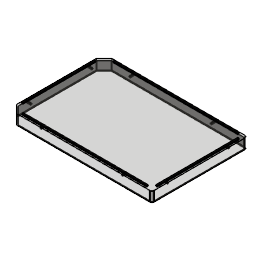
Container V3.4 (Assembly) (Autodesk Fusion 360 archive; units mm, degrees)
design "GREINER 96 WELL PLATE LID"
part number: 2026-02-05-10-27-23-618
Autodesk Fusion 360 part; units mm, degrees
(part 1 of 2)
sketch "Sketch1" plane through (0, 0, 0) normal (0, 0, 1) x (1, 0, 0)
  line L0 (61.42, -42.3) -> (-56.55, -42.3)
  line L1 (-63.55, -35.3) -> (-63.55, 35.3)
  line L2 (-56.55, 42.3) -> (61.42, 42.3)
  line L3 (63.55, 40.17) -> (63.55, -40.17)
  line L4 (63.55, -42.3) -> (-63.55, 42.3) construction
  line L5 (-63.55, -42.3) -> (63.55, 42.3) construction
  line L6 (-56.55, 42.3) -> (-63.55, 35.3)
  line L7 (0, -42.3) -> (0, 42.3) construction
  line L8 (63.55, 0) -> (-63.55, 0) construction
  line L9 (-56.55, -42.3) -> (-63.55, -35.3)
  arc A0 (63.55, 40.17) -> (61.42, 42.3) centre (61.42, 40.17) ccw
  arc A1 (61.42, -42.3) -> (63.55, -40.17) centre (61.42, -40.17) ccw
  dimension "d1" = 84.6
  dimension "d2" = 127.1
  dimension "d3" = 7
  dimension "d4" = 7
  dimension "d5" = 2.13
  constraint horizontal L0
  constraint perpendicular L0 L1
  constraint parallel L0 L2
  constraint parallel L1 L3
  constraint coincident L4 origin
  constraint coincident L5 origin
  constraint coincident L4.end L2
  constraint coincident L4.end L1
  constraint coincident L2 L7.end
  constraint perpendicular L2 L7
  constraint coincident L1 L8.end
  constraint perpendicular L1 L8
  constraint symmetric L2.start L8 L0.end
  constraint symmetric L1.end L8 L1.start
  constraint coincident L0 L7.start
  constraint coincident L3 L8.start
  constraint coincident L5.end L2
  constraint coincident L5.end L3
  constraint tangent L2 A0
  constraint tangent L3 A0
  constraint symmetric L8 L2.end L0.start
  constraint symmetric L8 L3.start L3.end
  constraint symmetric L8 A0 A1
  measures "d1" distance of L5.start L4.end
  measures "d2" distance of L4.end L5.end
  measures "d3" distance of L4.end L2.start
  measures "d4" distance of L4.end L1.end
  measures "d5" radius of A0
extrude "Extrude1" add sketch "Sketch1" against normal blind 9
sketch "Sketch2" plane through (0, 0, -9) normal (0, 0, -1) x (1, 0, 0)
  line L0 (61.42, 42.3) -> (-56.55, 42.3)
  line L1 (-56.55, 42.3) -> (-63.55, 35.3)
  line L2 (-63.55, 35.3) -> (-63.55, -35.3)
  line L3 (-63.55, -35.3) -> (-56.55, -42.3)
  line L4 (-56.55, -42.3) -> (61.42, -42.3)
  arc A0 (61.42, -42.3) -> (63.55, -40.17) centre (61.42, -40.17) ccw
  line L5 (63.55, -40.17) -> (63.55, 40.17)
  arc A1 (63.55, 40.17) -> (61.42, 42.3) centre (61.42, 40.17) ccw
  line L6 (61.42, -41.3) -> (-56.1358, -41.3)
  line L7 (-62.55, -34.8858) -> (-62.55, 34.8858)
  line L8 (-56.1358, 41.3) -> (61.42, 41.3)
  line L9 (62.55, 40.17) -> (62.55, -40.17)
  line L10 (62.55, -41.3) -> (-62.55, 41.3) construction
  line L11 (-62.55, -41.3) -> (62.55, 41.3) construction
  line L12 (-56.1358, 41.3) -> (-62.55, 34.8858)
  arc A2 (62.55, 40.17) -> (61.42, 41.3) centre (61.42, 40.17) ccw
  line L13 (63.55, 0) -> (-63.55, 0) construction
  line L14 (-56.1358, -41.3) -> (-62.55, -34.8858)
  arc A3 (61.42, -41.3) -> (62.55, -40.17) centre (61.42, -40.17) ccw
  dimension "d8" = 125.1
  dimension "d9" = 82.6
  dimension "d10" = 6.4142
  dimension "d11" = 6.4142
  dimension "d12" = 1
  dimension "d13" = 1.13
  constraint horizontal L6
  constraint perpendicular L6 L7
  constraint parallel L6 L8
  constraint parallel L7 L9
  constraint coincident L10 origin
  constraint coincident L11 origin
  constraint coincident L10.end L8
  constraint coincident L10.end L7
  constraint coincident L11.end L9
  constraint coincident L11.end L8
  constraint tangent L9 A2
  constraint tangent L8 A2
  constraint midpoint L5 L13.start
  constraint midpoint L2 L13.end
  constraint symmetric L8.start L13 L6.end
  constraint symmetric L7.end L13 L7.start
  constraint symmetric L9.start L13 L9.end
  constraint symmetric L8.end L13 L6.start
  constraint symmetric A2 L13 A3
  measures "d8" distance of L10.end L11.end
  measures "d9" distance of L11.start L10.end
  measures "d10" distance of L10.end L8.start
  measures "d11" distance of L10.end L7.end
  measures "d12" distance of L1 L12
  measures "d13" radius of A2
extrude "Extrude2" cut sketch "Sketch2" against normal blind 8 contours L6 L7 L8 L9 L12 A2 L14 A3
sketch "Sketch3" plane through (0, 0, -1) normal (0, 0, -1) x (1, 0, 0)
  line L0 (-56.1358, -41.3) -> (61.42, -41.3)
  arc A0 (61.42, -41.3) -> (62.55, -40.17) centre (61.42, -40.17) ccw
  line L1 (62.55, -40.17) -> (62.55, 40.17)
  arc A1 (62.55, 40.17) -> (61.42, 41.3) centre (61.42, 40.17) ccw
  line L2 (61.42, 41.3) -> (-56.1358, 41.3)
  line L3 (-56.1358, 41.3) -> (-62.55, 34.8858)
  line L4 (-62.55, 34.8858) -> (-62.55, -34.8858)
  line L5 (-62.55, -34.8858) -> (-56.1358, -41.3)
  line L6 (-62.55, 32.8642) -> (-35.55, 32.8642) construction
  line L7 (-35.55, 32.8642) -> (-35.55, 41.3) construction
  line L8 (-35.55, 41.3) -> (-36.55, 41.3)
  line L9 (-36.55, 41.3) -> (-36.55, 37.5)
  line L10 (-36.55, 37.5) -> (-35.55, 37.5)
  line L11 (-35.55, 37.5) -> (-35.55, 41.3)
  line L12 (-50.2731, 41.3) -> (-50.2731, 26.6) construction
  line L13 (-50.2731, 26.6) -> (-62.55, 26.6) construction
  line L14 (-62.55, 26.6) -> (-58.75, 26.6)
  line L15 (-58.75, 26.6) -> (-58.75, 27.6)
  line L16 (-58.75, 27.6) -> (-62.55, 27.6)
  line L17 (-62.55, 27.6) -> (-62.55, 26.6)
  line L18 (62.55, 0) -> (-62.55, 0) construction
  line L19 (-62.55, 30.673) -> (-62.55, 55) construction
  line L20 (62.55, 34.8173) -> (62.55, 55) construction
  line L21 (62.55, 55) -> (-62.55, 55) construction
  line L22 (0, 55) -> (0, -41.3) construction
  line L23 (62.55, 27.6) -> (62.55, 26.6)
  line L24 (62.55, 26.6) -> (58.75, 26.6)
  line L25 (58.75, 27.6) -> (62.55, 27.6)
  line L26 (58.75, 26.6) -> (58.75, 27.6)
  line L27 (36.55, 41.3) -> (36.55, 37.5)
  line L28 (35.55, 37.5) -> (35.55, 41.3)
  line L29 (36.55, 37.5) -> (35.55, 37.5)
  line L30 (35.55, 41.3) -> (36.55, 41.3)
  line L31 (62.55, -26.6) -> (58.75, -26.6)
  line L32 (58.75, -27.6) -> (62.55, -27.6)
  line L33 (58.75, -26.6) -> (58.75, -27.6)
  line L34 (35.55, -37.5) -> (35.55, -41.3)
  line L35 (36.55, -37.5) -> (35.55, -37.5)
  line L36 (36.55, -41.3) -> (36.55, -37.5)
  line L37 (62.55, -27.6) -> (62.55, -26.6)
  line L38 (35.55, -41.3) -> (36.55, -41.3)
  line L39 (-58.75, -26.6) -> (-58.75, -27.6)
  line L40 (-62.55, -26.6) -> (-58.75, -26.6)
  line L41 (-58.75, -27.6) -> (-62.55, -27.6)
  line L42 (-62.55, -27.6) -> (-62.55, -26.6)
  line L43 (-36.55, -37.5) -> (-35.55, -37.5)
  line L44 (-35.55, -37.5) -> (-35.55, -41.3)
  line L45 (-36.55, -41.3) -> (-36.55, -37.5)
  line L46 (-35.55, -41.3) -> (-36.55, -41.3)
  dimension "d16" = 27
  dimension "d17" = 3.8
  dimension "d18" = 1
  dimension "d19" = 14.7
  dimension "d20" = 3.8
  dimension "d21" = 1
  constraint coincident L4 L6.start
  constraint perpendicular L4 L6
  constraint coincident L2 L7.end
  constraint perpendicular L2 L7
  constraint horizontal L8
  constraint vertical L9
  constraint horizontal L10
  constraint vertical L11
  constraint coincident L2 L12.start
  constraint perpendicular L2 L12
  constraint coincident L4 L13.end
  constraint perpendicular L4 L13
  constraint horizontal L14
  constraint vertical L15
  constraint horizontal L16
  constraint vertical L17
  constraint midpoint L1 L18.start
  constraint midpoint L4 L18.end
  constraint coincident L4 L19.start
  constraint perpendicular L6 L19
  constraint coincident L1 L20.start
  constraint parallel L1 L20
  constraint perpendicular L19 L21
  constraint midpoint L21 L22.start
  constraint coincident L0 L22.end
  constraint perpendicular L0 L22
  constraint symmetric L7.end L22 L28.end
  constraint symmetric L8.end L22 L27.start
  constraint symmetric L9.end L22 L27.end
  constraint symmetric L10.end L22 L28.start
  constraint symmetric L13.end L22 L23.end
  constraint symmetric L14.end L22 L24.end
  constraint symmetric L15.end L22 L25.start
  constraint symmetric L16.end L22 L23.start
  constraint symmetric L7.end L18 L44.end
  constraint symmetric L8.end L18 L45.start
  constraint symmetric L9.end L18 L43.start
  constraint symmetric L10.end L18 L43.end
  constraint symmetric L13.end L18 L40.start
  constraint symmetric L14.end L18 L39.start
  constraint symmetric L15.end L18 L39.end
  constraint symmetric L16.end L18 L41.end
  constraint symmetric L18 L23.start L32.end
  constraint symmetric L18 L23.end L31.start
  constraint symmetric L18 L27.end L35.start
  constraint symmetric L18 L28.start L34.start
  constraint symmetric L18 L24.end L31.end
  constraint symmetric L18 L25.start L32.start
  constraint symmetric L18 L27.start L36.start
  constraint symmetric L18 L28.end L34.end
  measures "d16" distance of L6.start L6.end
  measures "d17" distance of L8.end L9.end
  measures "d18" distance of L9.end L10.end
  measures "d19" distance of L12.start L12.end
  measures "d20" distance of L15.end L16.end
  measures "d21" distance of L14.end L15.end
extrude "Extrude3" add sketch "Sketch3" along normal blind 1 contours L0 L43 L44 L45 L46 | L4 L39 L40 L41 L42 | L0 L34 L35 L36 L38 | L4 L14 L15 L16 L17 | L1 L31 L32 L33 L37 | L2 L8 L9 L10 L11 | L1 L23 L24 L25 L26 | L2 L27 L28 L29 L30
sketch "Sketch4" plane through (0, 0, 0) normal (0, 0, 1) x (-1, 0, 0)
  line L0 (56.55, 42.3) -> (-61.42, 42.3)
  arc A0 (-61.42, 42.3) -> (-63.55, 40.17) centre (-61.42, 40.17) ccw
  line L1 (-63.55, 40.17) -> (-63.55, -40.17)
  arc A1 (-63.55, -40.17) -> (-61.42, -42.3) centre (-61.42, -40.17) ccw
  line L2 (-61.42, -42.3) -> (56.55, -42.3)
  line L3 (56.55, -42.3) -> (63.55, -35.3)
  line L4 (63.55, -35.3) -> (63.55, 35.3)
  line L5 (63.55, 35.3) -> (56.55, 42.3)
  line L6 (-63.55, -34.3916) -> (-62.25, -34.3916) construction
  line L7 (-62.25, -34.3916) -> (-62.25, -36.4) construction
  line L8 (-60, -42.3) -> (-66.2, -42.3) construction
  line L9 (-63.55, -39.2433) -> (-63.55, -43.1) construction
  line L10 (-62.25, -36.4) -> (-60.95, -36.4)
  line L11 (-60.95, -36.4) -> (-60.95, 36.4)
  line L12 (-60.95, 36.4) -> (-62.25, 36.4)
  line L13 (-62.25, 36.4) -> (-62.25, -36.4)
  line L14 (-52.6219, -42.3) -> (-52.6219, -41) construction
  line L15 (-52.6219, -41) -> (-57.65, -41) construction
  line L16 (-57.65, -41) -> (53.05, -41)
  line L17 (53.05, -41) -> (53.05, -39.7)
  line L18 (53.05, -39.7) -> (-57.65, -39.7)
  line L19 (-57.65, -39.7) -> (-57.65, -41)
  line L20 (53.05, 39.7) -> (-57.65, 39.7)
  line L21 (-57.65, 41) -> (53.05, 41)
  line L22 (-57.65, 39.7) -> (-57.65, 41)
  line L23 (53.05, 41) -> (53.05, 39.7)
  line L24 (60.95, 0) -> (60.95, -32.3)
  line L25 (60.95, -32.3) -> (62.25, -32.3)
  line L26 (62.25, -32.3) -> (62.25, 0)
  line L27 (60.95, 0) -> (60.95, 32.3)
  line L28 (62.25, 32.3) -> (62.25, 0)
  line L29 (60.95, 32.3) -> (62.25, 32.3)
  line L30 (-63.55, 0) -> (60.95, 0) construction
  line L31 (62.25, 0) -> (63.55, 0) construction
  dimension "d24" = 1.3
  dimension "d25" = 5.9
  dimension "d26" = 72.8
  dimension "d27" = 1.3
  dimension "d28" = 1.3
  dimension "d29" = 5.9
  dimension "d30" = 1.3
  dimension "d31" = 110.7
  dimension "d32" = 32.3
  dimension "d33" = 1.3
  dimension "d34" = 1.3
  constraint coincident L1 L6.start
  constraint perpendicular L1 L6
  constraint perpendicular L6 L7
  constraint coincident L2 L8.start
  constraint parallel L2 L8
  constraint coincident L1 L9.start
  constraint perpendicular L2 L9
  constraint horizontal L10
  constraint vertical L11
  constraint horizontal L12
  constraint vertical L13
  constraint coincident L2 L14.start
  constraint perpendicular L2 L14
  constraint perpendicular L14 L15
  constraint horizontal L16
  constraint vertical L17
  constraint horizontal L18
  constraint vertical L19
  constraint midpoint L1 L30.start
  constraint midpoint L4 L31.end
  constraint symmetric L15.end L21.start L30
  constraint symmetric L16.end L21.end L30
  constraint symmetric L17.end L20.start L30
  constraint symmetric L18.end L20.end L30
  constraint vertical L24
  constraint horizontal L25
  constraint vertical L26
  constraint symmetric L24.end L27.end L30
  constraint symmetric L25.end L28.start L31
  constraint collinear L30 L31
  measures "d24" distance of L6.start L6.end
  measures "d25" distance of L7.end L8
  measures "d26" distance of L10.end L11.end
  measures "d27" distance of L7.end L10.end
  measures "d28" distance of L14.start L14.end
  measures "d29" distance of L9 L15.end
  measures "d30" distance of L15.end L18.end
  measures "d31" distance of L17.end L18.end
  measures "d32" distance of L24.start L24.end
  measures "d33" distance of L24.end L25.end
  measures "d34" distance of L4 L26
extrude "Extrude4" add sketch "Sketch4" along normal blind 1 contours L10 L11 L12 L13 | L16 L17 L18 L19 | L20 L21 L22 L23 | L24 L25 L26 L27 L28 L29
equation "d4 = d3"
equation "d11 = d10"

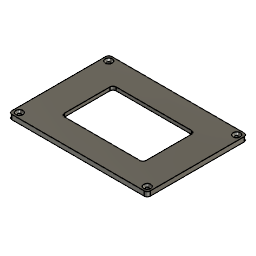
design "Lid V3.0"
part number: 2026-01-29-14-58-12-979
Autodesk Fusion 360 part; units mm, degrees
sketch "Sketch2" plane through (0, 0, 0) normal (0, 0, 1) x (1, 0, 0)
  line L0 (-48, 52) -> (124, 52)
  line L1 (128, 48) -> (128, -74)
  line L2 (124, -78) -> (-48, -78)
  line L3 (-52, -74) -> (-52, 48)
  circle A0 centre (-45, 45) radius 2.25
  line L4 (38, -78) -> (38, 52) construction
  line L5 (-52, -13) -> (128, -13) construction
  arc A1 (-48, 52) -> (-52, 48) centre (-48, 48) ccw
  circle A2 centre (121, 45) radius 2.25
  arc A3 (128, 48) -> (124, 52) centre (124, 48) ccw
  circle A4 centre (121, -71) radius 2.25
  arc A5 (124, -78) -> (128, -74) centre (124, -74) ccw
  circle A6 centre (-45, -71) radius 2.25
  arc A7 (-52, -74) -> (-48, -78) centre (-48, -74) ccw
  point P0 (-52, 52)
  point P1 (128, 52)
  dimension "d3" = 4.5
  dimension "d4" = 7
  dimension "d5" = 7
  dimension "d6" = 4
  dimension "d63" = 180
  dimension "d64" = 130
  constraint horizontal L0
  constraint vertical L1
  constraint horizontal L2
  constraint vertical L3
  constraint coincident L0 L4.end
  constraint coincident L3 L5.start
  constraint coincident P0 L0
  constraint coincident P0 L3
  constraint tangent L0 A1
  constraint tangent L3 A1
  constraint symmetric P0 L4 P1
  constraint symmetric A0 L4 A2
  constraint symmetric L4 L0.start L0.end
  constraint symmetric L4 L3.end L1.start
  constraint symmetric L4 A1 A3
  constraint coincident L1 L5.end
  constraint symmetric A0 L5 A6
  constraint symmetric L5 L0.start L2.end
  constraint symmetric L5 L3.end L3.start
  constraint symmetric L5 A1 A7
  constraint symmetric L5 L1.start L1.end
  constraint symmetric L5 L0.end L2.start
  constraint symmetric L5 A2 A4
  constraint symmetric L5 A3 A5
  constraint coincident L2 L4.start
  measures "d3" diameter of A0
  measures "d4" distance of L0 A0.centre
  measures "d5" distance of L3 A0.centre
  measures "d6" radius of A1
  measures "d63" distance of L1 L3
  measures "d64" distance of L0 L2
extrude "Extrude1" add sketch "Sketch2" along normal blind 6
sketch "Sketch3" plane through (0, 0, 0) normal (0, 0, -1) x (1, 0, 0)
  circle A0 centre (121, 71) radius 2.25
  circle A1 centre (-45, 71) radius 2.25
  circle A2 centre (-45, -45) radius 2.25
  circle A3 centre (121, -45) radius 2.25
  arc A4 (-52, -48) -> (-48, -52) centre (-48, -48) ccw
  line L0 (-48, -52) -> (124, -52)
  arc A5 (124, -52) -> (128, -48) centre (124, -48) ccw
  line L1 (128, -48) -> (128, 74)
  arc A6 (128, 74) -> (124, 78) centre (124, 74) ccw
  line L2 (124, 78) -> (-48, 78)
  arc A7 (-48, 78) -> (-52, 74) centre (-48, 74) ccw
  line L3 (-52, 74) -> (-52, -48)
  line L4 (38, 78) -> (38, -52) construction
  line L5 (128, 13) -> (-52, 13) construction
  line L6 (117.9494, -41.9494) -> (-41.9494, -41.9494) construction
  line L7 (-41.9494, -41.9494) -> (-41.9494, 67.9494) construction
  line L8 (-41.9494, 67.9494) -> (117.9494, 67.9494) construction
  line L9 (117.9494, 67.9494) -> (117.9494, -41.9494) construction
  line L10 (117.9494, -41.9494) -> (-41.9494, 67.9494) construction
  line L11 (-41.9494, -41.9494) -> (117.9494, 67.9494) construction
  line L12 (106.2459, -44.0839) -> (-30.2459, -44.0839)
  line L13 (-44.0839, -30.2459) -> (-44.0839, 56.2459)
  line L14 (-30.2459, 70.0839) -> (106.2459, 70.0839)
  line L15 (120.0839, 56.2459) -> (120.0839, -30.2459)
  line L16 (93.976, -25.9276) -> (-44.0839, 70.0839) construction
  line L17 (-38.2879, -33.8258) -> (83.9414, 41.199) construction
  line L18 (-39.8149, -30.2459) -> (-39.8149, 56.2459)
  line L19 (-30.2459, 65.8149) -> (106.2459, 65.8149)
  line L20 (115.8149, 56.2459) -> (115.8149, -30.2459)
  line L21 (103.0391, -31.1436) -> (-39.8149, 65.8149) construction
  line L22 (-35.6113, -30.989) -> (81.1607, 38.7921) construction
  arc A8 (-30.2459, 65.8149) -> (-39.8149, 56.2459) centre (-30.2459, 56.2459) ccw
  arc A9 (-30.2459, 70.0839) -> (-44.0839, 56.2459) centre (-30.2459, 56.2459) ccw
  arc A10 (115.8149, 56.2459) -> (106.2459, 65.8149) centre (106.2459, 56.2459) ccw
  arc A11 (120.0839, 56.2459) -> (106.2459, 70.0839) centre (106.2459, 56.2459) ccw
  arc A12 (-39.8149, -30.2459) -> (-30.2459, -39.8149) centre (-30.2459, -30.2459) ccw
  arc A13 (-44.0839, -30.2459) -> (-30.2459, -44.0839) centre (-30.2459, -30.2459) ccw
  arc A14 (106.2459, -39.8149) -> (115.8149, -30.2459) centre (106.2459, -30.2459) ccw
  arc A15 (106.2459, -44.0839) -> (120.0839, -30.2459) centre (106.2459, -30.2459) ccw
  line L23 (106.2459, -39.8149) -> (-30.2459, -39.8149)
  point P0 (38, 13)
  point P1 (38, 13)
  point P2 (38, 13)
  point P3 (38, 13)
  point P4 (38, 13)
  dimension "d25" = 159.8988
  dimension "d27" = 109.8988
  dimension "d28" = 2.1345
  dimension "d29" = 2.1345
  dimension "d30" = 2.1345
  dimension "d31" = 2.1345
  dimension "d44" = 9.569
  dimension "d45" = 13.838
  constraint midpoint L2 L4.start
  constraint midpoint L0 L4.end
  constraint midpoint L1 L5.start
  constraint midpoint L3 L5.end
  constraint midpoint L4 P4
  constraint coincident P4 P3
  constraint horizontal L6
  constraint perpendicular L6 L7
  constraint parallel L6 L8
  constraint parallel L7 L9
  constraint coincident L10 P4
  constraint coincident L11 P4
  constraint horizontal L12
  constraint perpendicular L12 L13
  constraint parallel L12 L14
  constraint parallel L13 L15
  constraint coincident L16 P4
  constraint coincident L17 P4
  constraint perpendicular L18 L23
  constraint parallel L19 L23
  constraint parallel L18 L20
  constraint coincident L21 P4
  constraint coincident L22 P4
  constraint coincident L21.end L19
  constraint coincident L21.end L18
  constraint tangent L19 A8
  constraint tangent L18 A8
  constraint coincident L16.end L14
  constraint coincident L16.end L13
  constraint tangent L14 A9
  constraint tangent L13 A9
  constraint symmetric L4 L19.start L19.end
  constraint symmetric L4 L18.end L20.start
  constraint symmetric L4 A8 A10
  constraint symmetric L4 L14.start L14.end
  constraint symmetric L4 L13.end L15.start
  constraint symmetric L4 A9 A11
  constraint symmetric L5 L19.start A12.end
  constraint symmetric L5 L18.end L18.start
  constraint symmetric L5 A8 A12
  constraint symmetric L5 L14.start L12.end
  constraint symmetric L5 L13.end L13.start
  constraint symmetric L5 A9 A13
  constraint symmetric L5 L19.end A14.start
  constraint symmetric L5 L20.start L20.end
  constraint symmetric L5 A10 A14
  constraint symmetric L5 L14.end L12.start
  constraint symmetric L5 L15.start L15.end
  constraint symmetric L5 A11 A15
  measures "d25" distance of L7.end L8.end
  measures "d27" distance of L6.end L7.end
  measures "d28" distance of L9 L15
  measures "d29" distance of L8 L14
  measures "d30" distance of L8 L19
  measures "d31" distance of L9 L20
  measures "d44" radius of A8
  measures "d45" radius of A9
extrude "Extrude4" add sketch "Sketch3" along normal blind 1.424 contours L12 L13 L14 L15 A9 A11 A13 A15
draft "Draft3" angle 10 neutral plane through (0, 0, -1.424) pull (0, 0, -1) 16 faces at (60.7486, -65.8149, -0.9493) (109.3756, -65.2886, -0.9493) (115.8149, -27.4153, -0.4747) (108.5019, 39.5452, -0.9493) (60.7486, 39.8149, -0.4747) (-38.5329, 35.0304, -0.9493) (-39.8149, -27.4153, -0.4747) (-32.5019, -65.5452, -0.9493) (-44.0839, 1.4153, -0.4747) (-35.389, 43.0927, -0.9493) (15.2514, 44.0839, -0.9493) (116.2609, 39.7952, -0.9493) (120.0839, 1.4153, -0.9493) (108.8648, -69.8338, -0.9493) (60.7486, -70.0839, -0.9493) (-44.0213, -57.5613, -0.4747)
sketch "Sketch5" plane through (0, 0, -1.424) normal (0, 0, -1) x (1, 0, 0)
  line L0 (-30.2459, 65.8149) -> (106.2459, 65.8149)
  line L1 (115.8149, 56.2459) -> (115.8149, -30.2459)
  line L2 (106.2459, -39.8149) -> (-30.2459, -39.8149)
  line L3 (-39.8149, -30.2459) -> (-39.8149, 56.2459)
  line L4 (106.2459, 70.0839) -> (-30.2459, 70.0839)
  line L5 (-44.0839, 56.2459) -> (-44.0839, -30.2459)
  line L6 (-30.2459, -44.0839) -> (106.2459, -44.0839)
  line L7 (120.0839, -30.2459) -> (120.0839, 56.2459)
  line L8 (38, 70.0839) -> (38, -44.0839) construction
  line L9 (120.0839, 13) -> (-44.0839, 13) construction
  line L10 (117.9494, -41.9494) -> (-41.9494, -41.9494) construction
  line L11 (-41.9494, -41.9494) -> (-41.9494, 67.9494) construction
  line L12 (-41.9494, 67.9494) -> (117.9494, 67.9494) construction
  line L13 (117.9494, 67.9494) -> (117.9494, -41.9494) construction
  line L14 (117.9494, -41.9494) -> (-41.9494, 67.9494) construction
  line L15 (-41.9494, -41.9494) -> (117.9494, 67.9494) construction
  line L16 (106.2459, -42.8839) -> (-30.2459, -42.8839)
  line L17 (-42.8839, -30.2459) -> (-42.8839, 56.2459)
  line L18 (-30.2459, 68.8839) -> (106.2459, 68.8839)
  line L19 (118.8839, 56.2459) -> (118.8839, -30.2459)
  line L20 (96.0985, -27.1411) -> (-42.8839, 68.8839) construction
  line L21 (-42.8839, -42.8839) -> (96.0985, 53.1411) construction
  line L22 (106.2459, -41.0149) -> (-30.2459, -41.0149)
  line L23 (-41.0149, -30.2459) -> (-41.0149, 56.2459)
  line L24 (117.0149, 56.2459) -> (117.0149, -30.2459)
  line L25 (95.1479, -26.0666) -> (-41.0149, 67.0149) construction
  line L26 (-41.0149, -41.0149) -> (95.1479, 52.0666) construction
  arc A0 (115.8149, 56.2459) -> (106.2459, 65.8149) centre (106.2459, 56.2459) ccw
  arc A1 (106.2459, -39.8149) -> (115.8149, -30.2459) centre (106.2459, -30.2459) ccw
  arc A2 (-39.8149, -30.2459) -> (-30.2459, -39.8149) centre (-30.2459, -30.2459) ccw
  arc A3 (-30.2459, 65.8149) -> (-39.8149, 56.2459) centre (-30.2459, 56.2459) ccw
  arc A4 (-44.0839, -30.2459) -> (-30.2459, -44.0839) centre (-30.2459, -30.2459) ccw
  arc A5 (106.2459, -44.0839) -> (120.0839, -30.2459) centre (106.2459, -30.2459) ccw
  arc A6 (120.0839, 56.2459) -> (106.2459, 70.0839) centre (106.2459, 56.2459) ccw
  arc A7 (-30.2459, 70.0839) -> (-44.0839, 56.2459) centre (-30.2459, 56.2459) ccw
  arc A8 (-30.2459, 67.0149) -> (-41.0149, 56.2459) centre (-30.2459, 56.2459) ccw
  arc A9 (-30.2459, 68.8839) -> (-42.8839, 56.2459) centre (-30.2459, 56.2459) ccw
  arc A10 (117.0149, 56.2459) -> (106.2459, 67.0149) centre (106.2459, 56.2459) ccw
  arc A11 (118.8839, 56.2459) -> (106.2459, 68.8839) centre (106.2459, 56.2459) ccw
  line L27 (-30.2459, 67.0149) -> (106.2459, 67.0149)
  arc A12 (106.2459, -41.0149) -> (117.0149, -30.2459) centre (106.2459, -30.2459) ccw
  arc A13 (106.2459, -42.8839) -> (118.8839, -30.2459) centre (106.2459, -30.2459) ccw
  arc A14 (-41.0149, -30.2459) -> (-30.2459, -41.0149) centre (-30.2459, -30.2459) ccw
  arc A15 (-42.8839, -30.2459) -> (-30.2459, -42.8839) centre (-30.2459, -30.2459) ccw
  point P0 (38, 13)
  point P1 (38, 13)
  point P2 (38, 13)
  dimension "d36" = 159.8988
  dimension "d37" = 109.8988
  dimension "d38" = 0.9345
  dimension "d39" = 0.9345
  dimension "d40" = 0.9345
  dimension "d41" = 0.9345
  dimension "d50" = 10.769
  dimension "d51" = 12.638
  constraint midpoint L4 L8.start
  constraint midpoint L6 L8.end
  constraint midpoint L7 L9.start
  constraint midpoint L5 L9.end
  constraint horizontal L10
  constraint perpendicular L10 L11
  constraint parallel L10 L12
  constraint parallel L11 L13
  constraint coincident L14 P2
  constraint coincident L15 P2
  constraint midpoint L8 P2
  constraint horizontal L16
  constraint perpendicular L16 L17
  constraint parallel L16 L18
  constraint parallel L17 L19
  constraint coincident L20 P2
  constraint coincident L21 P2
  constraint coincident P2 P1
  constraint horizontal L22
  constraint perpendicular L22 L23
  constraint parallel L22 L27
  constraint parallel L23 L24
  constraint coincident L25 P2
  constraint coincident L26 P2
  constraint coincident L26.start L23
  constraint coincident L26.start L22
  constraint coincident L21.start L17
  constraint coincident L21.start L16
  constraint coincident L25.end L27
  constraint coincident L25.end L23
  constraint tangent A8 L27
  constraint tangent L23 A8
  constraint coincident L20.end L18
  constraint coincident L20.end L17
  constraint tangent L18 A9
  constraint tangent L17 A9
  constraint symmetric L8 A8.start A10.end
  constraint symmetric L8 L23.end L24.start
  constraint symmetric L8 A8 A10
  constraint symmetric L8 L18.start L18.end
  constraint symmetric L8 L17.end L19.start
  constraint symmetric L8 A9 A11
  constraint symmetric L9 A10.end L22.start
  constraint symmetric L9 L24.start L24.end
  constraint symmetric L9 A10 A12
  constraint symmetric L9 L18.end L16.start
  constraint symmetric L9 L19.start L19.end
  constraint symmetric L9 A11 A13
  constraint symmetric L9 A8.start L22.end
  constraint symmetric L9 L23.end L23.start
  constraint symmetric L9 A8 A14
  constraint symmetric L9 L18.start L16.end
  constraint symmetric L9 L17.end L17.start
  constraint symmetric L9 A9 A15
  constraint coincident L23.start A14.start
  constraint coincident L17.start A15.start
  constraint coincident L22.end A14.end
  constraint coincident L16.end A15.end
  measures "d36" distance of L11.end L12.end
  measures "d37" distance of L10.end L11.end
  measures "d38" distance of L13 L19
  measures "d39" distance of L13 L24
  measures "d40" distance of L10 L16
  measures "d41" distance of L10 L22
  measures "d50" radius of A8
  measures "d51" radius of A9
extrude "Extrude6" cut sketch "Sketch5" against normal blind 1.424 contours L16 L17 L18 L19 A9 A11 A13 A15
extrude "Extrude7" cut 1 faces at (15.2514, -30.5213, 0) along direction (0, 0, 1) blind 0.5
sketch "Sketch6" plane through (0, 0, 0.5) normal (0, 0, -1) x (1, 0, 0)
  line L0 (106.2459, 65.5638) -> (-30.2459, 65.5638)
  arc A0 (-30.2459, 65.5638) -> (-39.5638, 56.2459) centre (-30.2459, 56.2459) ccw
  line L1 (-39.5638, 56.2459) -> (-39.5638, -30.2459)
  arc A1 (-39.5638, -30.2459) -> (-30.2459, -39.5638) centre (-30.2459, -30.2459) ccw
  line L2 (-30.2459, -39.5638) -> (106.2459, -39.5638)
  arc A2 (106.2459, -39.5638) -> (115.5638, -30.2459) centre (106.2459, -30.2459) ccw
  line L3 (115.5638, -30.2459) -> (115.5638, 56.2459)
  arc A3 (115.5638, 56.2459) -> (106.2459, 65.5638) centre (106.2459, 56.2459) ccw
  line L4 (38, 65.5638) -> (38, -39.5638) construction
  line L5 (-39.5638, 13) -> (115.5638, 13) construction
  line L6 (92, -25.5) -> (-16, -25.5)
  line L7 (-20, -21.5) -> (-20, 47.5)
  line L8 (-16, 51.5) -> (92, 51.5)
  line L9 (96, 47.5) -> (96, -21.5)
  line L10 (96, -25.5) -> (-20, 51.5) construction
  line L11 (-20, -25.5) -> (96, 51.5) construction
  arc A4 (-16, 51.5) -> (-20, 47.5) centre (-16, 47.5) ccw
  arc A5 (96, 47.5) -> (92, 51.5) centre (92, 47.5) ccw
  arc A6 (92, -25.5) -> (96, -21.5) centre (92, -21.5) ccw
  arc A7 (-20, -21.5) -> (-16, -25.5) centre (-16, -21.5) ccw
  point P0 (38, 13)
  dimension "d58" = 116
  dimension "d59" = 77
  dimension "d68" = 4
  dimension "d69" = 4
  dimension "d70" = 4
  dimension "d71" = 4
  constraint midpoint L0 L4.start
  constraint midpoint L2 L4.end
  constraint midpoint L1 L5.start
  constraint midpoint L3 L5.end
  constraint horizontal L6
  constraint perpendicular L6 L7
  constraint parallel L6 L8
  constraint parallel L7 L9
  constraint coincident L10 P0
  constraint coincident L11 P0
  constraint midpoint L5 P0
  constraint coincident L10.end L8
  constraint coincident L10.end L7
  constraint tangent L8 A4
  constraint tangent L7 A4
  constraint coincident L11.end L8
  constraint coincident L11.end L9
  constraint tangent L8 A5
  constraint tangent L9 A5
  constraint coincident L10.start L9
  constraint coincident L10.start L6
  constraint tangent L9 A6
  constraint tangent L6 A6
  constraint coincident L11.start L7
  constraint coincident L11.start L6
  constraint tangent L7 A7
  constraint tangent L6 A7
  measures "d58" distance of L10.end L11.end
  measures "d59" distance of L11.start L10.end
  measures "d68" radius of A4
  measures "d69" radius of A5
  measures "d70" radius of A6
  measures "d71" radius of A7
extrude "Extrude8" cut sketch "Sketch6" against normal blind 1.1 contours L6 L7 L8 L9 A4 A5 A6 A7
sketch "Sketch7" plane through (0, 0, 1.6) normal (0, 0, -1) x (1, 0, 0)
  line L0 (92, 51.5) -> (-16, 51.5)
  line L1 (-20, 47.5) -> (-20, -21.5)
  line L2 (-16, -25.5) -> (92, -25.5)
  line L3 (96, -21.5) -> (96, 47.5)
  line L4 (38, 51.5) -> (38, -25.5) construction
  line L5 (96, 13) -> (-20, 13) construction
  line L6 (87, -20.5) -> (-11, -20.5)
  line L7 (-15, -16.5) -> (-15, 42.5)
  line L8 (-11, 46.5) -> (87, 46.5)
  line L9 (91, 42.5) -> (91, -16.5)
  line L10 (91, -20.5) -> (-15, 46.5) construction
  line L11 (-15, -20.5) -> (91, 46.5) construction
  arc A0 (-16, 51.5) -> (-20, 47.5) centre (-16, 47.5) ccw
  arc A1 (-20, -21.5) -> (-16, -25.5) centre (-16, -21.5) ccw
  arc A2 (92, -25.5) -> (96, -21.5) centre (92, -21.5) ccw
  arc A3 (96, 47.5) -> (92, 51.5) centre (92, 47.5) ccw
  arc A4 (-11, 46.5) -> (-15, 42.5) centre (-11, 42.5) ccw
  arc A5 (91, 42.5) -> (87, 46.5) centre (87, 42.5) ccw
  arc A6 (87, -20.5) -> (91, -16.5) centre (87, -16.5) ccw
  arc A7 (-15, -16.5) -> (-11, -20.5) centre (-11, -16.5) ccw
  point P0 (38, 13)
  dimension "d62" = 106
  dimension "d65" = 67
  dimension "d72" = 4
  dimension "d73" = 4
  dimension "d74" = 4
  dimension "d75" = 4
  constraint midpoint L0 L4.start
  constraint midpoint L2 L4.end
  constraint midpoint L3 L5.start
  constraint midpoint L1 L5.end
  constraint horizontal L6
  constraint perpendicular L6 L7
  constraint parallel L6 L8
  constraint parallel L7 L9
  constraint coincident L10 P0
  constraint coincident L11 P0
  constraint midpoint L4 P0
  constraint coincident L10.end L8
  constraint coincident L10.end L7
  constraint tangent L8 A4
  constraint tangent L7 A4
  constraint coincident L11.end L9
  constraint coincident L11.end L8
  constraint tangent L9 A5
  constraint tangent L8 A5
  constraint coincident L10.start L9
  constraint coincident L10.start L6
  constraint tangent L9 A6
  constraint tangent L6 A6
  constraint coincident L11.start L6
  constraint coincident L11.start L7
  constraint tangent L6 A7
  constraint tangent L7 A7
  measures "d62" distance of L10.end L11.end
  measures "d65" distance of L11.start L10.end
  measures "d72" radius of A4
  measures "d73" radius of A5
  measures "d74" radius of A6
  measures "d75" radius of A7
extrude "Extrude9" cut sketch "Sketch7" against normal blind 8.4 contours L6 L7 L8 L9 A4 A5 A6 A7
sketch "Sketch9" plane through (0, 0, 6) normal (0, 0, 1) x (-1, 0, 0)
  line L0 (15, 42.5) -> (15, -16.5)
  arc A0 (11, -20.5) -> (15, -16.5) centre (11, -16.5) ccw
  line L1 (11, -20.5) -> (-87, -20.5)
  arc A1 (-91, -16.5) -> (-87, -20.5) centre (-87, -16.5) ccw
  line L2 (-91, -16.5) -> (-91, 42.5)
  arc A2 (-87, 46.5) -> (-91, 42.5) centre (-87, 42.5) ccw
  line L3 (-87, 46.5) -> (11, 46.5)
  arc A3 (15, 42.5) -> (11, 46.5) centre (11, 42.5) ccw
  circle A4 centre (-121, 71) radius 2.25
  circle A5 centre (-121, -45) radius 2.25
  circle A6 centre (45, 71) radius 2.25
  circle A7 centre (45, -45) radius 2.25
  arc A8 (48, -52) -> (52, -48) centre (48, -48) ccw
  line L4 (52, -48) -> (52, 74)
  arc A9 (52, 74) -> (48, 78) centre (48, 74) ccw
  line L5 (48, 78) -> (-124, 78)
  arc A10 (-124, 78) -> (-128, 74) centre (-124, 74) ccw
  line L6 (-128, 74) -> (-128, -48)
  arc A11 (-128, -48) -> (-124, -52) centre (-124, -48) ccw
  line L7 (-124, -52) -> (48, -52)
  line L8 (45, -47.25) -> (45, -42.75) construction
  line L9 (42.75, -45) -> (47.25, -45) construction
  circle A12 centre (45, -45) radius 4
  line L10 (-38, -52) -> (-38, 78) construction
  line L11 (-128, 13) -> (52, 13) construction
  circle A13 centre (-121, -45) radius 4
  circle A14 centre (45, 71) radius 4
  circle A15 centre (-121, 71) radius 4
  dimension "d91" = 8
  constraint coincident A7 L8.start
  constraint coincident A7 L8.end
  constraint vertical L8
  constraint coincident A7 L9.start
  constraint coincident A7 L9.end
  constraint perpendicular L8 L9
  constraint concentric A7 A12
  constraint midpoint L7 L10.start
  constraint midpoint L5 L10.end
  constraint midpoint L6 L11.start
  constraint midpoint L4 L11.end
  constraint symmetric A12 L10 A13
  constraint symmetric A12 L11 A14
  constraint symmetric L11 A13 A15
  measures "d91" diameter of A12
sketch "Sketch10" plane through (0, 0, 0.5) normal (0, 0, -1) x (1, 0, 0)
  line L0 (-20, -21.5) -> (-20, 47.5)
  arc A0 (-16, 51.5) -> (-20, 47.5) centre (-16, 47.5) ccw
  line L1 (-16, 51.5) -> (92, 51.5)
  arc A1 (96, 47.5) -> (92, 51.5) centre (92, 47.5) ccw
  line L2 (96, 47.5) -> (96, -21.5)
  arc A2 (92, -25.5) -> (96, -21.5) centre (92, -21.5) ccw
  line L3 (92, -25.5) -> (-16, -25.5)
  arc A3 (-20, -21.5) -> (-16, -25.5) centre (-16, -21.5) ccw
  line L4 (106.2459, 65.5638) -> (-30.2459, 65.5638)
  arc A4 (-30.2459, 65.5638) -> (-39.5638, 56.2459) centre (-30.2459, 56.2459) ccw
  line L5 (-39.5638, 56.2459) -> (-39.5638, -30.2459)
  arc A5 (-39.5638, -30.2459) -> (-30.2459, -39.5638) centre (-30.2459, -30.2459) ccw
  line L6 (-30.2459, -39.5638) -> (106.2459, -39.5638)
  arc A6 (106.2459, -39.5638) -> (115.5638, -30.2459) centre (106.2459, -30.2459) ccw
  line L7 (115.5638, -30.2459) -> (115.5638, 56.2459)
  arc A7 (115.5638, 56.2459) -> (106.2459, 65.5638) centre (106.2459, 56.2459) ccw
  line L8 (38, 65.5638) -> (38, -39.5638) construction
  line L9 (115.5638, 13) -> (-39.5638, 13) construction
  line L10 (38, 13) -> (-24.24, 13) construction
  line L11 (-23.09, 11) -> (-25.39, 11)
  line L12 (-25.39, 11) -> (-25.39, 15)
  line L13 (-25.39, 15) -> (-23.09, 15)
  line L14 (-23.09, 15) -> (-23.09, 11)
  line L15 (-23.09, 11) -> (-25.39, 15) construction
  line L16 (-25.39, 11) -> (-23.09, 15) construction
  line L17 (38, 13) -> (38, 54) construction
  line L18 (40, 52.85) -> (36, 52.85)
  line L19 (36, 52.85) -> (36, 55.15)
  line L20 (36, 55.15) -> (40, 55.15)
  line L21 (40, 55.15) -> (40, 52.85)
  line L22 (40, 52.85) -> (36, 55.15) construction
  line L23 (36, 52.85) -> (40, 55.15) construction
  line L24 (99.09, 15) -> (99.09, 11)
  line L25 (101.39, 15) -> (99.09, 15)
  line L26 (101.39, 11) -> (101.39, 15)
  line L27 (99.09, 11) -> (101.39, 11)
  line L28 (40, -26.85) -> (36, -26.85)
  line L29 (40, -29.15) -> (40, -26.85)
  line L30 (36, -29.15) -> (40, -29.15)
  line L31 (36, -26.85) -> (36, -29.15)
  point P0 (-24.24, 13)
  point P1 (38, 54)
  dimension "d97" = 62.24
  dimension "d98" = 2.3
  dimension "d99" = 4
  dimension "d100" = 41
  dimension "d101" = 2.3
  dimension "d102" = 4
  constraint midpoint L4 L8.start
  constraint midpoint L6 L8.end
  constraint midpoint L7 L9.start
  constraint midpoint L5 L9.end
  constraint midpoint L9 L10.start
  constraint perpendicular L8 L10
  constraint horizontal L11
  constraint perpendicular L11 L12
  constraint parallel L11 L13
  constraint parallel L12 L14
  constraint coincident L15 P0
  constraint coincident L16 P0
  constraint coincident P0 L10.end
  constraint perpendicular L9 L17
  constraint horizontal L18
  constraint perpendicular L18 L19
  constraint parallel L18 L20
  constraint parallel L19 L21
  constraint coincident L22 P1
  constraint coincident L23 P1
  constraint coincident P1 L17.end
  constraint symmetric L8 L11.start L24.end
  constraint symmetric L8 L11.end L26.start
  constraint symmetric L8 L12.end L25.start
  constraint symmetric L8 L13.end L24.start
  constraint symmetric L9 L18.start L28.start
  constraint symmetric L9 L18.end L28.end
  constraint symmetric L9 L19.end L30.start
  constraint symmetric L9 L20.end L29.start
  measures "d97" distance of L10.start P0
  measures "d98" distance of L12.end L13.end
  measures "d99" distance of L11.end L12.end
  measures "d100" distance of L10.start P1
  measures "d101" distance of L18.start L20.end
  measures "d102" distance of L19.end L20.end
extrude "Extrude12" add sketch "Sketch10" along normal blind 4.2 contours L11 L12 L13 L14 | L18 L19 L20 L21 | L24 L25 L26 L27 | L28 L29 L30 L31
chamfer "Chamfer2" distance 2.4 angle 45 4 edges at (-47.0977, 45.8136, 6) (118.9023, 45.8136, 6) (118.9023, -70.1864, 6) (-47.0977, -70.1864, 6) measured on face at (111.574, -3.1667, 6) measured on face at (111.574, -3.1667, 6) measured on face at (111.574, -3.1667, 6) measured on face at (111.574, -3.1667, 6)
equation "d3 = Bolt_Diam + 0.5 mm"
equation "ORingDiameter = 1.78 mm" comment "Diamter of the O ring"
equation "ORingInnerDiameter = 170 mm" comment "Inner diamter of the o ring bore"
equation "d25 = ( ORingPerimeter - 100 mm ) / 4 + 50 mm"
equation "ORingPerimeter = 2 * 3.1412 * ( ( ORingInnerDiameter / 2 ) + ORingDiameter / 2 )"
equation "d27 = ( ORingPerimeter - 100 mm ) / 4"
equation "d28 = ( ( ORingDiameter * 1.05 ) / 2 ) + 1.2 mm"
equation "d29 = ( ( ORingDiameter * 1.05 ) / 2 ) + 1.2 mm"
equation "d30 = ( ( ORingDiameter * 1.05 ) / 2 ) + 1.2 mm"
equation "d31 = ( ( ORingDiameter * 1.05 ) / 2 ) + 1.2 mm"
equation "d32 = ORingDiameter * 0.8"
equation "d36 = ( ORingPerimeter - 100 mm ) / 4 + 50 mm"
equation "d37 = ( ORingPerimeter - 100 mm ) / 4"
equation "d38 = ( ORingDiameter * 1.05 ) / 2"
equation "d39 = ( ORingDiameter * 1.05 ) / 2"
equation "d40 = ( ORingDiameter * 1.05 ) / 2"
equation "d41 = ( ORingDiameter * 1.05 ) / 2"
equation "d44 = ( ORingDiameter ) * 6 + ORingDiameter * 0.05 - 1.2 mm"
equation "d45 = ( ORingDiameter ) * 6 + ( ORingDiameter * 1.1 ) + 1.2 mm"
equation "d50 = ( ORingDiameter ) * 6 + ORingDiameter * 0.05 - 0.0 mm"
equation "d51 = ( ORingDiameter ) * 6 + ORingDiameter * 1.1 + 0 mm"
equation "d52 = -( ORingDiameter * 0.8 )"
equation "PanelWidth = 77 mm"
equation "PanelLength = 116 mm"
equation "d58 = PanelLength"
equation "d59 = PanelWidth"
equation "d62 = PanelLength - 10 mm"
equation "d65 = PanelWidth - 10 mm"
equation "d91 = Bolt_Head_Diam"
equation "Bolt_Diam = 4 mm" comment "Diameter of the bolt"
equation "Bolt_Head_Height = 2.3 mm" comment "Height of th ebolt head"
equation "Bolt_Head_Diam = 8 mm" comment "Diamter of the bolt head"
equation "d106 = Bolt_Head_Height + 0.1 mm"

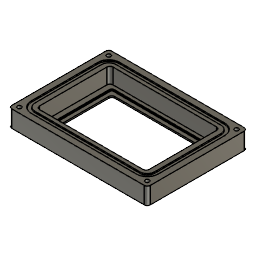
design "Base V3.0"
part number: 2026-01-30-14-30-51-369
Autodesk Fusion 360 part; units mm, degrees
sketch "Sketch1" plane through (0, 0, 0) normal (0, 0, 1) x (1, 0, 0)
  line L0 (86, -65) -> (-86, -65)
  line L1 (-90, -61) -> (-90, 61)
  line L2 (-86, 65) -> (86, 65)
  line L3 (90, 61) -> (90, -61)
  line L4 (90, -65) -> (-90, 65) construction
  line L5 (-90, -65) -> (90, 65) construction
  arc A0 (-86, 65) -> (-90, 61) centre (-86, 61) ccw
  arc A1 (90, 61) -> (86, 65) centre (86, 61) ccw
  arc A2 (86, -65) -> (90, -61) centre (86, -61) ccw
  arc A3 (-90, -61) -> (-86, -65) centre (-86, -61) ccw
  circle A4 centre (-83, 58) radius 2.6
  line L6 (0, 65) -> (0, -65) construction
  line L7 (90, 0) -> (-90, 0) construction
  circle A5 centre (83, 58) radius 2.6
  circle A6 centre (83, -58) radius 2.6
  circle A7 centre (-83, -58) radius 2.6
  dimension "d1" = 180
  dimension "d2" = 130
  dimension "d26" = 4
  dimension "d27" = 4
  dimension "d28" = 4
  dimension "d29" = 4
  dimension "d30" = 5.2
  dimension "d31" = 7
  dimension "d32" = 7
  constraint horizontal L0
  constraint perpendicular L0 L1
  constraint parallel L0 L2
  constraint parallel L1 L3
  constraint coincident L4 origin
  constraint coincident L5 origin
  constraint coincident L4.end L2
  constraint coincident L4.end L1
  constraint tangent L2 A0
  constraint tangent L1 A0
  constraint coincident L5.end L3
  constraint coincident L5.end L2
  constraint tangent L3 A1
  constraint tangent L2 A1
  constraint coincident L4.start L3
  constraint coincident L4.start L0
  constraint tangent L3 A2
  constraint tangent L0 A2
  constraint coincident L5.start L1
  constraint coincident L5.start L0
  constraint tangent L1 A3
  constraint tangent L0 A3
  constraint midpoint L2 L6.start
  constraint midpoint L0 L6.end
  constraint midpoint L3 L7.start
  constraint midpoint L1 L7.end
  constraint symmetric A4 L6 A5
  constraint symmetric A4 L7 A7
  constraint symmetric L7 A5 A6
  measures "d1" distance of L4.end L5.end
  measures "d2" distance of L5.start L4.end
  measures "d26" radius of A0
  measures "d27" radius of A1
  measures "d28" radius of A2
  measures "d29" radius of A3
  measures "d30" diameter of A4
  measures "d31" distance of L2 A4.centre
  measures "d32" distance of L1 A4.centre
extrude "Extrude1" add sketch "Sketch1" along normal blind 22
sketch "Sketch2" plane through (0, 0, 22) normal (0, 0, 1) x (-1, 0, 0)
  line L0 (-86, -65) -> (86, -65)
  line L1 (90, -61) -> (90, 61)
  line L2 (86, 65) -> (-86, 65)
  line L3 (-90, 61) -> (-90, -61)
  line L4 (-67.2, 47.75) -> (67.2, 47.75)
  line L5 (71.2, 43.75) -> (71.2, -43.75)
  line L6 (67.2, -47.75) -> (-67.2, -47.75)
  line L7 (-71.2, -43.75) -> (-71.2, 43.75)
  line L8 (-71.2, 47.75) -> (71.2, -47.75) construction
  line L9 (71.2, 47.75) -> (-71.2, -47.75) construction
  arc A0 (86, -65) -> (90, -61) centre (86, -61) ccw
  arc A1 (90, 61) -> (86, 65) centre (86, 61) ccw
  arc A2 (-86, 65) -> (-90, 61) centre (-86, 61) ccw
  arc A3 (-90, -61) -> (-86, -65) centre (-86, -61) ccw
  circle A4 centre (83, 58) radius 2.6
  circle A5 centre (-83, 58) radius 2.6
  circle A6 centre (-83, -58) radius 2.6
  circle A7 centre (83, -58) radius 2.6
  arc A8 (67.2, -47.75) -> (71.2, -43.75) centre (67.2, -43.75) ccw
  arc A9 (-71.2, -43.75) -> (-67.2, -47.75) centre (-67.2, -43.75) ccw
  arc A10 (71.2, 43.75) -> (67.2, 47.75) centre (67.2, 43.75) ccw
  arc A11 (-67.2, 47.75) -> (-71.2, 43.75) centre (-67.2, 43.75) ccw
  dimension "d5" = 142.4
  dimension "d6" = 95.5
  dimension "d52" = 4
  dimension "d53" = 4
  dimension "d54" = 4
  dimension "d55" = 4
  constraint horizontal L4
  constraint perpendicular L4 L5
  constraint parallel L4 L6
  constraint parallel L5 L7
  constraint coincident L8 origin
  constraint coincident L9 origin
  constraint coincident L8.end L6
  constraint coincident L8.end L5
  constraint tangent L6 A8
  constraint tangent L5 A8
  constraint coincident L9.end L6
  constraint coincident L9.end L7
  constraint tangent L6 A9
  constraint tangent L7 A9
  constraint coincident L9.start L5
  constraint coincident L9.start L4
  constraint tangent L5 A10
  constraint tangent L4 A10
  constraint coincident L8.start L7
  constraint coincident L8.start L4
  constraint tangent L7 A11
  constraint tangent L4 A11
  measures "d5" distance of L8.end L9.end
  measures "d6" distance of L9.start L8.end
  measures "d52" radius of A8
  measures "d53" radius of A9
  measures "d54" radius of A10
  measures "d55" radius of A11
extrude "Extrude2" cut sketch "Sketch2" against normal blind 20 contours L4 L5 L6 L7 A8 A9 A10 A11
sketch "Sketch3" plane through (0, 0, 22) normal (0, 0, 1) x (-1, 0, 0)
  line L0 (71.2, 43.75) -> (71.2, -43.75)
  line L1 (67.2, -47.75) -> (-67.2, -47.75)
  line L2 (-71.2, -43.75) -> (-71.2, 43.75)
  line L3 (-67.2, 47.75) -> (67.2, 47.75)
  line L4 (-86, -65) -> (86, -65)
  line L5 (90, -61) -> (90, 61)
  line L6 (86, 65) -> (-86, 65)
  line L7 (-90, 61) -> (-90, -61)
  line L8 (-79.9494, 54.9494) -> (79.9494, 54.9494) construction
  line L9 (79.9494, 54.9494) -> (79.9494, -54.9494) construction
  line L10 (79.9494, -54.9494) -> (-79.9494, -54.9494) construction
  line L11 (-79.9494, -54.9494) -> (-79.9494, 54.9494) construction
  line L12 (-79.9494, 54.9494) -> (79.9494, -54.9494) construction
  line L13 (79.9494, 54.9494) -> (-79.9494, -54.9494) construction
  line L14 (77.8149, 43.2459) -> (77.8149, -43.2459)
  line L15 (68.2459, -52.8149) -> (-68.2459, -52.8149)
  line L16 (-77.8149, -43.2459) -> (-77.8149, 43.2459)
  line L17 (-69.6267, 47.2574) -> (77.8149, -52.8149) construction
  line L18 (70.6619, 45.6619) -> (-70.6619, -45.6619) construction
  line L19 (-68.2459, 57.0839) -> (68.2459, 57.0839)
  line L20 (82.0839, 43.2459) -> (82.0839, -43.2459)
  line L21 (68.2459, -57.0839) -> (-68.2459, -57.0839)
  line L22 (-82.0839, -43.2459) -> (-82.0839, 43.2459)
  line L23 (-72.3401, 50.3077) -> (82.0839, -57.0839) construction
  line L24 (73.5309, 48.5309) -> (-73.5309, -48.5309) construction
  arc A0 (68.2459, -52.8149) -> (77.8149, -43.2459) centre (68.2459, -43.2459) ccw
  arc A1 (68.2459, -57.0839) -> (82.0839, -43.2459) centre (68.2459, -43.2459) ccw
  line L25 (0, -65) -> (0, 65) construction
  line L26 (-90, 0) -> (90, 0) construction
  arc A2 (-77.8149, -43.2459) -> (-68.2459, -52.8149) centre (-68.2459, -43.2459) ccw
  arc A3 (-82.0839, -43.2459) -> (-68.2459, -57.0839) centre (-68.2459, -43.2459) ccw
  arc A4 (-68.2459, 52.8149) -> (-77.8149, 43.2459) centre (-68.2459, 43.2459) ccw
  arc A5 (-68.2459, 57.0839) -> (-82.0839, 43.2459) centre (-68.2459, 43.2459) ccw
  arc A6 (77.8149, 43.2459) -> (68.2459, 52.8149) centre (68.2459, 43.2459) ccw
  arc A7 (82.0839, 43.2459) -> (68.2459, 57.0839) centre (68.2459, 43.2459) ccw
  line L27 (-68.2459, 52.8149) -> (68.2459, 52.8149)
  arc A8 (86, -65) -> (90, -61) centre (86, -61) ccw
  arc A9 (90, 61) -> (86, 65) centre (86, 61) ccw
  arc A10 (-86, 65) -> (-90, 61) centre (-86, 61) ccw
  arc A11 (-90, -61) -> (-86, -65) centre (-86, -61) ccw
  circle A12 centre (83, 58) radius 2.6
  circle A13 centre (-83, 58) radius 2.6
  circle A14 centre (-83, -58) radius 2.6
  circle A15 centre (83, -58) radius 2.6
  arc A16 (71.2, 43.75) -> (67.2, 47.75) centre (67.2, 43.75) ccw
  arc A17 (67.2, -47.75) -> (71.2, -43.75) centre (67.2, -43.75) ccw
  arc A18 (-71.2, -43.75) -> (-67.2, -47.75) centre (-67.2, -43.75) ccw
  arc A19 (-67.2, 47.75) -> (-71.2, 43.75) centre (-67.2, 43.75) ccw
  dimension "d9" = 159.8988
  dimension "d15" = 109.8988
  dimension "d16" = 2.1345
  dimension "d17" = 2.1345
  dimension "d18" = 2.1345
  dimension "d19" = 2.1345
  dimension "d20" = 9.569
  dimension "d21" = 13.838
  constraint horizontal L8
  constraint perpendicular L8 L9
  constraint parallel L8 L10
  constraint parallel L9 L11
  constraint coincident L12 origin
  constraint coincident L13 origin
  constraint parallel L15 L27
  constraint parallel L14 L16
  constraint coincident L17 origin
  constraint coincident L18 origin
  constraint horizontal L19
  constraint perpendicular L19 L20
  constraint parallel L19 L21
  constraint parallel L20 L22
  constraint coincident L23 origin
  constraint coincident L24 origin
  constraint coincident L17.end L15
  constraint coincident L17.end L14
  constraint tangent L15 A0
  constraint tangent L14 A0
  constraint coincident L23.end L21
  constraint coincident L23.end L20
  constraint tangent L21 A1
  constraint tangent L20 A1
  constraint midpoint L4 L25.start
  constraint midpoint L6 L25.end
  constraint midpoint L7 L26.start
  constraint midpoint L5 L26.end
  constraint symmetric L15.start L25 L15.end
  constraint symmetric L14.end L25 L16.start
  constraint symmetric A0 L25 A2
  constraint symmetric L21.start L25 L21.end
  constraint symmetric L20.end L25 L22.start
  constraint symmetric A1 L25 A3
  constraint symmetric L15.start L26 A6.end
  constraint symmetric L14.end L26 L14.start
  constraint symmetric A0 L26 A6
  constraint symmetric L21.start L26 L19.end
  constraint symmetric L20.end L26 L20.start
  constraint symmetric A1 L26 A7
  constraint symmetric L26 L15.end A4.start
  constraint symmetric L26 L16.start L16.end
  constraint symmetric L26 A2 A4
  constraint symmetric L26 L21.end L19.start
  constraint symmetric L26 L22.start L22.end
  constraint symmetric L26 A3 A5
  measures "d9" distance of L8.start L8.end
  measures "d15" distance of L8 L10
  measures "d16" distance of L11 L16
  measures "d17" distance of L10 L15
  measures "d18" distance of L11 L22
  measures "d19" distance of L10 L21
  measures "d20" radius of A0
  measures "d21" radius of A1
extrude "Extrude3" cut sketch "Sketch3" against normal blind 1.424 contours L19 L20 L21 L22 A1 A3 A5 A7
draft "Draft1" angle 10 neutral plane through (0, 0, 20.576) pull (0, 0, 1) 16 faces at (-77.8149, -14.4153, 21.5253) (-71.8024, 52.1295, 21.0507) (-22.7486, 52.8149, 21.5253) (72.6307, 51.7512, 21.0507) (77.8149, 14.4153, 21.5253) (73.0304, -51.5329, 21.0507) (22.7486, -52.8149, 21.5253) (-77.1295, -46.8024, 21.0507) (-82.0839, -14.4153, 21.5253) (-76.2727, -54.518, 21.0507) (-22.7486, -57.0839, 21.0507) (82.0213, -44.5613, 21.0507) (82.0839, 14.4153, 21.5253) (77.7952, 53.2609, 21.0507) (22.7486, 57.0839, 21.0507) (-76.8, 54.1233, 21.0507)